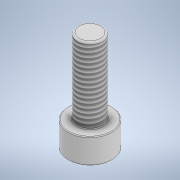
# Autodesk Inventor part: MM-MMount_to_Motor-Bolt
Saved by Autodesk Inventor 2020 (Build 240168000, 168)
## iProperties
Created: 2020-02-26
Part Number: MM-MMount_to_Motor-Bolt
Material: Generic
Document SubType Name: Modeling
Designer: Vitaliy
Density: 1 g/cm^3
Appearance: Default
Author: Vitaliy
Autodesk Inventor part; units mm, degrees
ref_plane "YZ Plane" through (0, 0, 0) normal (1, 0, 0) x (0, 1, 0)
ref_plane "XZ Plane" through (0, 0, 0) normal (0, 1, 0) x (-1, 0, 0)
ref_plane "XY Plane" through (0, 0, 0) normal (0, 0, 1) x (1, 0, 0)
sketch "Sketch1" plane through (0, 0, 0) normal (0, 1, 0) x (-1, 0, 0)
  circle A0 centre (0, 0) radius 3.5
  dimension "d0" = 7
  constraints: 1 centre point, 1 coincident
  measures "d0" diameter of A0
extrude "Extrusion1" add sketch "Sketch1" along normal blind 4
sketch "Sketch2" plane through (0, 4, 0) normal (0, 1, 0) x (1, 0, 0)
  circle A0 centre (0, 0) radius 2
  dimension "d3" = 4
  constraints: 1 centre point, 1 coincident
  measures "d3" diameter of A0
extrude "Extrusion2" add sketch "Sketch2" along normal blind 12
sketch "Sketch3" plane through (0, 0, 0) normal (0, -1, 0) x (1, 0, 0)
  line L0 (-1.7321, 0) -> (-0.866, 1.5)
  line L1 (-0.866, 1.5) -> (0.866, 1.5)
  line L2 (0.866, 1.5) -> (1.7321, 0)
  line L3 (1.7321, 0) -> (0.866, -1.5)
  line L4 (0.866, -1.5) -> (-0.866, -1.5)
  line L5 (-0.866, -1.5) -> (-1.7321, 0)
  point P0 (0, 0)
  point P1 (0, 0)
  dimension "d6" = 3
  constraints: 12 end point, 1 coincident, 13 other
  measures "d6" distance between parallel lines of L2 L5
extrude "Extrusion3" cut sketch "Sketch3" against normal blind 2.7
thread "Thread1" size "M4x0.7" class "6g" standard "ISO Metric profile" length 24
fillet "Fillet1" radius 0.3 1 edges at (-2, 16, 0)
fillet "Fillet2" radius 0.125 3 edges at (-2, 4, 0) (3.5, 4, 0) (3.5, 0, 0)
fillet "Fillet3" radius 0.05 13 edges at (-1.299, 0, -0.75) (-1.299, 0, 0.75) (0, 0, 1.5) (1.299, 0, 0.75) (1.299, 0, -0.75) (0.866, 1.35, -1.5) (0, 0, -1.5) (-1.299, 2.7, -0.75) (-1.299, 2.7, 0.75) (0, 2.7, 1.5) (1.299, 2.7, 0.75) (1.299, 2.7, -0.75) (0, 2.7, -1.5)
body "Solid1"
